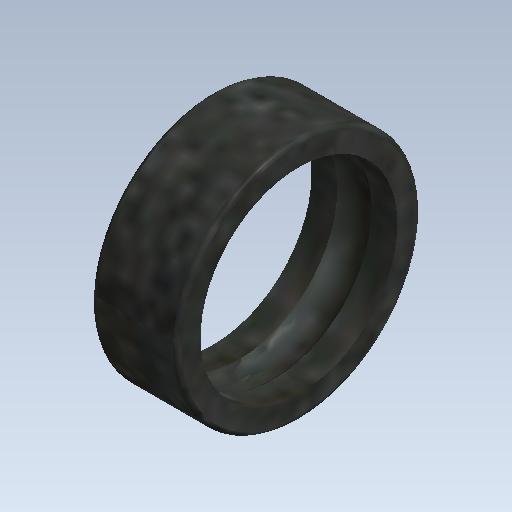
# Autodesk Inventor part: 606 Outer Ring
Saved by Autodesk Inventor 2021 (Build 250183000, 183)
## iProperties
Part Number: 606 Outer Ring
Material: Steel
Catalog Web Link: www.cadenas.de
Description: open_type_OR-
Vendor: NSK_RB
Document SubType Name: Modeling
Designer: partserver
Manufacturer: NSK_RB
Mass: 3.37457 g
Surface Area: 7.41349 cm^2
Volume: 0.429881 cm^3
Density: 7.85 g/cm^3
Appearance: Plate
Category: PARTsolutions
Company: NSK_RB
PSOL_IDENT_0: {$CADENAS_DATA\23d-libs\nsk_rb\roller_bearings\deep_groove_bb\exstra_small_miniatur_bb\metric_design
PSOL_IDENT_1: \open_type_or_2.prj},176 {VTYP=3D},{NB=606 Outer Ring},{LINA=606 Outer Ring},{NN=open_type_OR},{DATE=
PSOL_IDENT_2: 10.04.2020 04:57:45},{GEOMDATE=04.01.2008 00:00:00},{VERSION=},{LINEID=1680},{WBVAR=},{WBNUMERIC=}
PSOL_IDENT_3: {NB=606 Outer Ring},{LINA=606 Outer Ring},{KT=DUMMY},{IDNR=},{STAN=Standard},{ORDER=606},{SD=6.0},{X=
PSOL_IDENT_4: 6.0},{DI1=8.92},{SDE1=13.75},{D=17},{DD=17},{B=6.0},{B1=0.0},{R=0.30},{R1=0.00},{CR1=2260},{COR1=835
PSOL_IDENT_5: },{CR2=231},{COR2=85.0},{LG=38000},{LO=45000},{DA=8.0},{DB=0.0},{DA1=15.0},{DB1=0.0},{RA=0.30},{RB=0
PSOL_IDENT_6: .00},{MASS=5.97},{SC=1}
NB: 606 Outer Ring
NN: open_type_OR
NBSYN: $ORDER. Outer Ring
LINA: 606 Outer Ring
CATALOG: NSK Rolling Bearing
STAN: Standard
ORDER: 606
SD: 6
X: 6
DI1: 8.92
SDE1: 13.75
D: 17
DD: 17
B: 6
B1: 0
R: 0.3
R1: 0
CR1: 2260
COR1: 835
CR2: 231
COR2: 85
LG: 38000
LO: 45000
DA: 8
DB: 0
DA1: 15
DB1: 0
RA: 0.3
RB: 0
MASS: 5.97
SC: 1
SUPPLIER: NSK_RB
ARTICLENO: 606 Outer Ring
BOMINFO: 606 Outer Ring
CREATOR: CADENAS GmbH
Title: 606 Outer Ring
Author: Cadenas PARTsolutions
Autodesk Inventor part; units mm, degrees
sketch "Sketch_1" plane through (0, 0, 0) normal (0, 0, 1) x (1, 0, 0)
  line L0 (6, 0) -> (0, 0)
  line L1 (0, 6.875) -> (1.793, 6.875)
  arc A0 (4.207, 6.875) -> (1.793, 6.875) centre (3, 5.75) ccw
  line L2 (4.207, 6.875) -> (6, 6.875)
  line L3 (6, 6.875) -> (6, 8.2)
  arc A1 (6, 8.2) -> (5.7, 8.5) centre (5.7, 8.2) ccw
  line L4 (5.7, 8.5) -> (0.3, 8.5)
  arc A2 (0.3, 8.5) -> (0, 8.2) centre (0.3, 8.2) ccw
  line L5 (0, 8.2) -> (0, 6.875)
  constraints: 12 end point, 6 point on circle, 3 centre point
revolve "Revolution1" add sketch "Sketch_1" angle 360 about axis through (6, 0, 0) along (1, 0, 0)
ref_plane "ip_ot_or_XY" through (0, 0, 0) normal (1, 0, 0) x (0, 0, -1)
ref_plane "ip_ot_or_YZ" through (0, 0, 0) normal (0, 0, -1) x (0, 1, 0)
ref_plane "ip_ot_or_ZX" through (0, 0, 0) normal (0, 1, 0) x (1, 0, 0)
body "Solid1"
